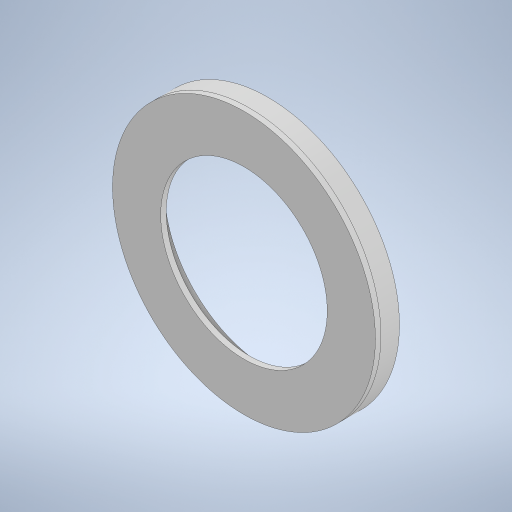
# Autodesk Inventor part: Ball_Gearing_Workaroung
Saved by Autodesk Inventor 2023 (Build 270158000, 158)
## iProperties
Created: 2022-09-14
Part Number: Ball_Gearing_Workaroung
Material: Generic
Document SubType Name: Modeling
Designer: Windows10
Density: 1 g/cm^3
Appearance: Default
Author: Windows10
Autodesk Inventor part; units mm, degrees
ref_plane "YZ Plane" through (0, 0, 0) normal (1, 0, 0) x (0, 1, 0)
ref_plane "XZ Plane" through (0, 0, 0) normal (0, 1, 0) x (-1, 0, 0)
ref_plane "XY Plane" through (0, 0, 0) normal (0, 0, 1) x (1, 0, 0)
sketch "Sketch1" plane through (0, 0, 0) normal (0, 0, 1) x (1, 0, 0)
  circle A0 centre (0, 0) radius 2.485
  circle A1 centre (0, 0) radius 1.65
  circle A2 centre (10.4407, 0) radius 5.6
  circle A3 centre (10.4407, 0) radius 7.1
  dimension "d0" = 4.97
  dimension "d3" = 3.3
  dimension "d4" = 11.2
  dimension "d5" = 1.5
  constraints: 4 centre point, 3 coincident
  measures "d0" diameter of A0
  measures "d3" diameter of A1
  measures "d4" diameter of A2
  measures "d5" radial gap between concentric circles of A3 A2
extrude "Extrusion1" add sketch "Sketch1" along normal blind 4 contours A0
extrude "Extrusion2" add sketch "Sketch1" along normal blind 1 separate body contours A3
sketch "Sketch2" plane through (10.4407, 0, 1) normal (0, 0, 1) x (1, 0, 0)
  circle A0 centre (0, 0) radius 7.1 projected
  circle A1 centre (0, 0) radius 5.6 projected
  circle A2 centre (0, 0) radius 4.5
  point P0 (-10.4407, 0)
  dimension "d8" = 9
  constraints: 1 centre point, 1 coincident
  measures "d8" diameter of A2
extrude "Extrusion4" add sketch "Sketch2" along normal blind 0.3 separate body contours A0 | A1
body "Solid1"
body "Solid2"
body "Solid4"
